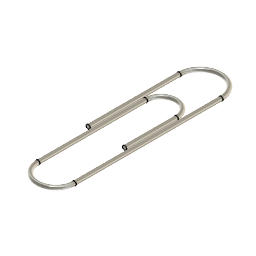
clip (Autodesk Fusion 360 design; units mm, degrees)
part number: 2025-09-17-13-23-31-424
Autodesk Fusion 360 part; units mm, degrees
sketch "Sketch1" plane through (0, 0, 0) normal (0, 0, 1) x (1, 0, 0)
  line L0 (0, 0) -> (0, 16.25)
  line L1 (0, 16.25) -> (7.5, 16.25) construction
  line L2 (7.5, 16.25) -> (7.5, -10)
  line L3 (7.5, -10) -> (1, -10) construction
  line L4 (1, -10) -> (1, 9.25)
  line L5 (1, 9.25) -> (6.5, 9.25) construction
  line L6 (6.5, 9.25) -> (6.5, 0)
  arc A0 (7.5, 16.25) -> (0, 16.25) centre (3.75, 16.25) ccw
  arc A1 (1, -10) -> (7.5, -10) centre (4.25, -10) ccw
  arc A2 (6.5, 9.25) -> (1, 9.25) centre (3.75, 9.25) ccw
  dimension "d1" = 16.25
  dimension "d2" = 90
  dimension "d3" = 7.5
  dimension "d4" = 90
  dimension "d5" = 26.25
  dimension "d6" = 90
  dimension "d7" = 6.5
  dimension "d8" = 90
  dimension "d9" = 19.25
  dimension "d10" = 90
  dimension "d11" = 5.5
  dimension "d12" = 90
  dimension "d13" = 9.25
  constraint vertical L0
  constraint coincident L0.start origin
  constraint tangent L0 A0
  constraint tangent L2 A1
  constraint tangent L4 A2
  measures "d1" distance of L0.start L0.end
  measures "d2" angle of L0 L1
  measures "d3" distance of L0.end L1.end
  measures "d4" angle of L1 L2
  measures "d5" distance of L1.end L2.end
  measures "d6" angle of L2 L3
  measures "d7" distance of L2.end L3.end
  measures "d8" angle of L3 L4
  measures "d9" distance of L3.end L4.end
  measures "d10" angle of L4 L5
  measures "d11" distance of L4.end L5.end
  measures "d12" angle of L5 L6
  measures "d13" distance of L5.end L6.end
sketch "Sketch2" plane through (0, 0, 0) normal (0, 1, 0) x (1, 0, 0)
  circle A0 centre (0, 0) radius 0.375
  dimension "d14" = 0.75
  constraint coincident A0.centre origin
  measures "d14" diameter of A0
sweep "Sweep1" add profiles "Sketch2" path "Sketch1" along L0 A0 L2 A1 L4 A2 L6 section 1
